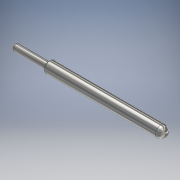
# Autodesk Inventor part: Tommy Bar
Saved by Autodesk Inventor 2018 (Build 220112000, 112)
## iProperties
Created: 2019-08-31
Part Number: Tommy Bar
Material: Generic
Document SubType Name: Modeling
Designer: HP
Density: 1 g/cm^3
Appearance: Chrome - Polished
Author: HP
Autodesk Inventor part; units mm, degrees
ref_plane "YZ Plane" through (0, 0, 0) normal (1, 0, 0) x (0, 1, 0)
ref_plane "XZ Plane" through (0, 0, 0) normal (0, 1, 0) x (-1, 0, 0)
ref_plane "XY Plane" through (0, 0, 0) normal (0, 0, 1) x (1, 0, 0)
sketch "Sketch1" plane through (0, 0, 0) normal (0, 0, 1) x (1, 0, 0)
  line L0 (0, 0) -> (275, 0)
  line L1 (275, 0) -> (275, 10)
  line L2 (0, 0) -> (0, 6)
  line L3 (0, 6) -> (62, 6)
  line L4 (62, 6) -> (66, 10)
  line L5 (275, 10) -> (66, 10)
  dimension "d0" = 275
  dimension "d1" = 10
  dimension "d2" = 6
  dimension "d3" = 62
  dimension "d5" = 135
  constraints: 12 end point, 2 horizontal, 1 parallel, 1 perpendicular, 1 vertical
  measures "d0" distance of L0.start L0.end
  measures "d1" distance of L0.end L1.end
  measures "d2" distance of L0.start L2.end
  measures "d3" distance of L2.end L3.end
  measures "d5" angle of L4 L3
revolve "Revolution1" add sketch "Sketch1" angle 360 about axis through (0, 0, 0) along (1, 0, 0)
fillet "Fillet1" [suppressed]
fillet "Fillet2" radius 10 1 edges at (275, -10, 0)
fillet "Fillet3" radius 6 1 edges at (0, -6, 0)
body "Solid1"
